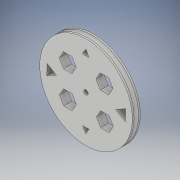
# Autodesk Inventor part: Hew O Ring
Saved by Autodesk Inventor 2017 (Build 210142000, 142)
## iProperties
Created: 2016-09-29
Part Number: Hew O Ring
Material: Generic
Document SubType Name: Modeling
Designer: Student
Density: 1 g/cm^3
Appearance: Default
Author: Student
Autodesk Inventor part; units mm, degrees
ref_plane "YZ Plane" through (0, 0, 0) normal (1, 0, 0) x (0, 1, 0)
ref_plane "XZ Plane" through (0, 0, 0) normal (0, 1, 0) x (-1, 0, 0)
ref_plane "XY Plane" through (0, 0, 0) normal (0, 0, 1) x (1, 0, 0)
sketch "Sketch1" plane through (0, 0, 0) normal (0, 0, 1) x (1, 0, 0)
  circle A0 centre (0, 0) radius 36.9824
  dimension "d17" = 73.9648
  constraints: 1 centre point
  measures "d17" diameter of A0
extrude "Extrusion1" add sketch "Sketch1" along normal mid plane 6.35
sketch "Sketch4" plane through (0, 0, 0) normal (1, 0, 0) x (0, 1, 0)
  circle A0 centre (36.9824, 0) radius 1.7653
  line L0 (36.9824, -3.175) -> (36.9824, 3.175) construction
  line L1 (36.9824, -3.175) -> (36.9824, 3.175)
  line L2 (36.9824, -3.175) -> (36.9824, 3.175) projected
  line L3 (0, -6.8515) -> (0, 6.9022)
  point P0 (0, 0)
  dimension "d5" = 3.5306
  constraints: 4 end point, 2 point on line, 1 centre point, 1 coincident, 1 midpoint, 1 vertical
  measures "d5" diameter of A0
revolve "Revolution1" cut sketch "Sketch4" angle 360 about axis through (0, 0, -6.8515) along (0, 0, 1)
sketch "Sketch5" plane through (0, -10.4797, 3.175) normal (0, 0, 1) x (1, 0, 0)
  line L0 (11.3113, 29.5816) -> (18.1134, 29.6722)
  line L1 (18.1134, 29.6722) -> (21.5928, 23.8267)
  line L2 (21.5928, 23.8267) -> (18.2702, 17.8907)
  line L3 (18.2702, 17.8907) -> (11.4682, 17.8001)
  line L4 (11.4682, 17.8001) -> (7.9887, 23.6456)
  line L5 (7.9887, 23.6456) -> (11.3113, 29.5816)
  line L6 (-18.0537, 29.5853) -> (-11.2517, 29.6759)
  line L7 (-11.2517, 29.6759) -> (-7.7722, 23.8304)
  line L8 (-7.7722, 23.8304) -> (-11.0948, 17.8944)
  line L9 (-11.0948, 17.8944) -> (-17.8969, 17.8038)
  line L10 (-17.8969, 17.8038) -> (-21.3763, 23.6493)
  line L11 (-21.3763, 23.6493) -> (-18.0537, 29.5853)
  line L12 (-17.916, 3.9729) -> (-11.114, 4.0635)
  line L13 (-11.114, 4.0635) -> (-7.6345, -1.782)
  line L14 (-7.6345, -1.782) -> (-10.9571, -7.718)
  line L15 (-10.9571, -7.718) -> (-17.7592, -7.8086)
  line L16 (-17.7592, -7.8086) -> (-21.2386, -1.9631)
  line L17 (-21.2386, -1.9631) -> (-17.916, 3.9729)
  line L18 (11.6578, 3.5557) -> (18.4598, 3.6463)
  line L19 (18.4598, 3.6463) -> (21.9393, -2.1992)
  line L20 (21.9393, -2.1992) -> (18.6167, -8.1352)
  line L21 (18.6167, -8.1352) -> (11.8146, -8.2257)
  line L22 (11.8146, -8.2257) -> (8.3352, -2.3803)
  line L23 (8.3352, -2.3803) -> (11.6578, 3.5557)
  line L24 (-23.7615, 10.4722) -> (-31.2466, 6.34)
  line L25 (-31.2466, 6.34) -> (-31.0827, 14.8884)
  line L26 (-31.0827, 14.8884) -> (-23.7615, 10.4722)
  line L27 (23.8373, 10.4722) -> (31.6292, 14.9709)
  line L28 (31.6292, 14.9709) -> (31.6292, 5.9736)
  line L29 (31.6292, 5.9736) -> (23.8373, 10.4722)
  line L30 (2.3663, 35.8446) -> (-2.7917, 35.9364)
  line L31 (-2.7917, 35.9364) -> (-0.1332, 40.3574)
  line L32 (-0.1332, 40.3574) -> (2.3663, 35.8446)
  line L33 (2.3663, -13.8498) -> (-0.0945, -18.246)
  line L34 (-0.0945, -18.246) -> (-2.6714, -13.9168)
  line L35 (-2.6714, -13.9168) -> (2.3663, -13.8498)
  point P0 (0, 10.4797)
  point P1 (14.7908, 23.7362)
  point P2 (-14.5743, 23.7399)
  point P3 (-14.4366, -1.8725)
  point P4 (15.1372, -2.2897)
  point P5 (-28.6969, 10.5669)
  point P6 (29.0319, 10.4722)
  point P7 (-0.1862, 37.3795)
  point P8 (-0.1332, -15.3375)
  constraints: 72 end point, 80 other
extrude "Extrusion3" cut sketch "Sketch5" against normal through all
sketch "Sketch6" plane through (0, -10.4797, 3.175) normal (0, 0, 1) x (1, 0, 0)
  circle A0 centre (0, 10.4797) radius 1.524
  circle A1 centre (0, 10.4797) radius 36.9824 projected
  dimension "d9" = 3.048
  constraints: 1 centre point, 1 coincident
  measures "d9" diameter of A0
extrude "Extrusion4" cut sketch "Sketch6" against normal through all contours A0
sketch "Sketch9" plane through (0, 0, -3.175) normal (0, 0, -1) x (-1, 0, 0)
  circle A0 centre (0, 0) radius 4.445
  circle A1 centre (0, 0) radius 1.524 projected
  dimension "d14" = 8.89
  constraints: 3 coincident, 1 centre point
  measures "d14" diameter of A0
extrude "Extrusion5" cut sketch "Sketch9" against normal blind 3.175
sketch "Sketch11" plane through (0, -10.4797, -3.175) normal (0, 0, -1) x (-1, 0, 0)
  arc A0 (6.84, 6.338) -> (19.5394, 8.1514) centre (2.6508, 81.0506) ccw
  arc A1 (19.5394, 8.1514) -> (19.5394, 12.8081) centre (19, 10.4797) ccw
  arc A2 (19.5394, 12.8081) -> (6.84, 14.6214) centre (2.6508, -60.0911) ccw
  arc A3 (4.1417, 17.3197) -> (2.3283, 30.0191) centre (-70.5709, 13.1305) ccw
  arc A4 (2.3283, 30.0191) -> (-2.3283, 30.0191) centre (0, 29.4797) ccw
  arc A5 (-2.3283, 30.0191) -> (-4.1417, 17.3197) centre (70.5709, 13.1305) ccw
  arc A6 (-6.84, 14.6214) -> (-19.5394, 12.8081) centre (-2.6508, -60.0911) ccw
  arc A7 (-19.5394, 12.8081) -> (-19.5394, 8.1514) centre (-19, 10.4797) ccw
  arc A8 (-19.5394, 8.1514) -> (-6.84, 6.338) centre (-2.6508, 81.0506) ccw
  arc A9 (-4.1417, 3.6397) -> (-2.3283, -9.0597) centre (70.5709, 7.8289) ccw
  arc A10 (-2.3283, -9.0597) -> (2.3283, -9.0597) centre (0, -8.5203) ccw
  arc A11 (2.3283, -9.0597) -> (4.1417, 3.6397) centre (-70.5709, 7.8289) ccw
  circle A12 centre (0, 20.7297) radius 0.4953
  circle A13 centre (0, 23.7197) radius 0.4953
  circle A14 centre (0, 26.4497) radius 0.4953
  circle A15 centre (0, 17.8197) radius 0.5
  circle A16 centre (0, 10.4797) radius 2.9464
  circle A17 centre (-7.34, 10.4797) radius 0.5
  circle A18 centre (-10.25, 10.4797) radius 0.4953
  circle A19 centre (-13.24, 10.4797) radius 0.4953
  circle A20 centre (-15.97, 10.4797) radius 0.4953
  circle A21 centre (7.34, 10.4797) radius 0.5
  circle A22 centre (10.25, 10.4797) radius 0.4953
  circle A23 centre (13.24, 10.4797) radius 0.4953
  circle A24 centre (15.97, 10.4797) radius 0.4953
  circle A25 centre (0, 3.1397) radius 0.5
  circle A26 centre (0, 0.2297) radius 0.4953
  circle A27 centre (0, -2.7603) radius 0.4953
  circle A28 centre (0, -5.4903) radius 0.4953
  line L0 (-4.1417, 17.3197) -> (-6.84, 14.6214)
  line L1 (4.1417, 17.3197) -> (6.84, 14.6214)
  line L2 (6.84, 6.338) -> (4.1417, 3.6397)
  line L3 (-6.84, 6.338) -> (-4.1417, 3.6397)
  constraints: 29 centre point, 24 point on circle, 8 end point, 1 perpendicular
extrude "Extrusion6" cut sketch "Sketch11" against normal blind 2.032 contours L2 A11 A10 A9 L3 A8 A7 A6 L0 A5 A4 A3 L1 A2 A1 A0 | A12 | A13 | A14 | A15 | A17 | A18 | A19 | A20 | A21 | A22 | A23 | A24 | A25 | A26 | A27 | A28
sketch "Sketch12" plane through (0, 0, 3.175) normal (0, 0, 1) x (1, 0, 0)
  circle A0 centre (0, 0) radius 1.778
  dimension "d20" = 3.556
  constraints: 1 centre point, 1 coincident
  measures "d20" diameter of A0
extrude "Extrusion7" cut sketch "Sketch12" against normal blind 1.27
body "Solid1"
